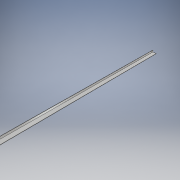
# Autodesk Inventor part: Profile-T#01
Saved by Autodesk Inventor 2018 (Build 220112000, 112)
## iProperties
Created: 2025-02-16
Part Number: Profile-T#01
Material: Všeobecné
Document SubType Name: Modeling
Designer: Jozko Mrkvicka
Density: 1 g/cm^3
Appearance: Výchozí
Author: Jozko Mrkvicka
Autodesk Inventor part; units mm, degrees
ref_plane "YZ Plane" through (0, 0, 0) normal (1, 0, 0) x (0, 1, 0)
ref_plane "XZ Plane" through (0, 0, 0) normal (0, 1, 0) x (-1, 0, 0)
ref_plane "XY Plane" through (0, 0, 0) normal (0, 0, 1) x (1, 0, 0)
sketch "Náčrt1" plane through (0, 0, 0) normal (0, 0, 1) x (1, 0, 0)
  line L0 (0, 0) -> (30, 0)
  line L1 (30, 0) -> (30, 2)
  line L2 (30, 2) -> (16, 2)
  line L3 (16, 2) -> (16, 30)
  line L4 (16, 30) -> (14, 30)
  line L5 (14, 30) -> (14, 2)
  line L6 (14, 2) -> (0, 2)
  line L7 (0, 2) -> (0, 0)
  dimension "d0" = 30
  dimension "d1" = 2
  dimension "d2" = 14
  dimension "d3" = 28
  dimension "d4" = 2
  constraints: 16 end point, 4 perpendicular, 2 point on line, 1 horizontal, 1 parallel, 1 vertical
  measures "d0" distance of L0.start L0.end
  measures "d1" distance of L0.end L1.end
  measures "d2" distance of L1.end L2.end
  measures "d3" distance of L2.end L3.end
  measures "d4" distance of L3.end L4.end
extrude "Vysunutí1" add sketch "Náčrt1" along normal blind 1200
sketch "Náčrt2" plane through (16, 2, 0) normal (0, 1, 0) x (1, 0, 0)
  line L0 (0, 0) -> (0, -1200) projected
  line L1 (14, -1200) -> (0, -1200) projected
  circle A0 centre (7, -1185) radius 1.5
  line L2 (14, 0) -> (14, -1200) projected
  line L3 (14, -600) -> (0, -600)
  circle A1 centre (7, -15) radius 1.5
  point P0 (-16, 0)
  dimension "d7" = 15
  dimension "d8" = 3
  constraints: 2 centre point, 2 end point, 2 midpoint, 1 symmetric about line, 1 other
  measures "d7" distance from line of A0.centre L1
  measures "d8" diameter of A0
extrude "Vysunutí2" cut sketch "Náčrt2" against normal up to next contours A0 | A1
equation "\"d0\" = width_A"
equation "\"d2\" = -0.5 * thickness + 0.5 * width_A"
equation "\"d3\" = width_B - thickness"
equation "\"d4\" = thickness"
equation "\"d5\" = length"
equation "\"d7\" = 0.5 * gSquareProfile_Width_Rack"
equation "\"width_A\" = 30"
equation "\"width_B\" = 30"
equation "\"thickness\" = 2"
equation "\"length\" = gRack_Cpu_Length"
equation "\"gSquareProfile_Width_Rack\" = 30"
equation "\"gRack_Cpu_Length\" = 1200"
